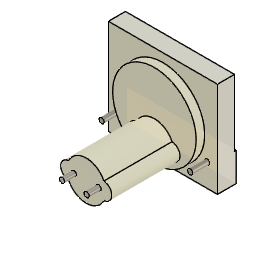
cpu usage panel v51 (Autodesk Fusion 360 archive; units mm, degrees)
design "galvanometer"
Autodesk Fusion 360 part; units mm, degrees
sketch "Sketch1" plane through (0, 0, 0) normal (0, 1, 0) x (1, 0, 0)
  line L0 (32, -28) -> (-32, -28)
  line L1 (-32, -28) -> (-32, 28)
  line L2 (-32, 28) -> (32, 28)
  line L3 (32, 28) -> (32, -28)
  line L4 (32, -28) -> (-32, 28) construction
  circle A0 centre (0, 1.5) radius 24.5
  line L5 (0, 1.5) -> (0, 0) construction
  line L6 (26, 14.5) -> (-26, 14.5) construction
  line L7 (0, 0) -> (0, 14.5) construction
  circle A1 centre (-26, 14.5) radius 1.5
  line L8 (32, 11) -> (-32, 11)
  circle A2 centre (0, 14.5) radius 11.5
  circle A3 centre (-7.25, 14.5) radius 1.5
  circle A4 centre (-10, 14.5) radius 5
  circle A5 centre (26, 14.5) radius 1.5
  circle A6 centre (10, 14.5) radius 5
  circle A7 centre (7.25, 14.5) radius 1.5
  dimension "d1" = 64
  dimension "d2" = 56
  dimension "d3" = 49
  dimension "d4" = 1.5
  dimension "d5" = 52
  dimension "d6" = 14.5
  dimension "d7" = 3
  dimension "d14" = 17
  dimension "d18" = 23
  dimension "d19" = 3
  dimension "d20" = 7.25
  dimension "d26" = 10
  dimension "d27" = 10
  constraint horizontal L0
  constraint vertical L1
  constraint horizontal L2
  constraint vertical L3
  constraint midpoint L5.end L4
  constraint coincident A0.centre L5.start
  constraint coincident L5.end L7.start
  constraint vertical L5
  constraint horizontal L6
  constraint perpendicular L6 L7
  constraint midpoint L6 L7.end
  constraint coincident L6.end A1.centre
  constraint coincident L3 L8.start
  constraint coincident L1 L8.end
  constraint perpendicular L1 L8
  constraint coincident L7 A2.centre
  constraint coincident L7.end A2.centre
  constraint coincident L6 A3.centre
  constraint symmetric L7 A1 A5
  constraint symmetric L7 A3 A7
  constraint symmetric L7 A4 A6
  constraint coincident L6 A4.centre
  measures "d1" distance of L0.start L0.end
  measures "d2" distance of L0.end L1.end
  measures "d3" diameter of A0
  measures "d4" distance of L5.end A0.centre
  measures "d5" distance of L6.start L6.end
  measures "d6" distance of L5.end L7.end
  measures "d7" diameter of A1
  measures "d14" distance of L2 L8
  measures "d18" diameter of A2
  measures "d19" diameter of A3
  measures "d20" distance of L7.end A3.centre
  measures "d26" diameter of A4
  measures "d27" distance of L7.end A4.centre
extrude "Extrude1" add sketch "Sketch1" along normal blind 10 contours L0 L1 L3 A0 L8 | L1 L2 L3 A0 L8 | A0 L8 A2 A6 | A0 L8 A2 A4 A6 | A0 L8 A2 A4 | L8 A2 A4 A6 | L8 A2 A6 | L8 A2 A6 | L8 A2 A4 | L8 A2 A4 | L8 A2 A6 | L8 A2 A4 | L8 A2 A6 | L8 A2 A4 A6 | L8 A2 A4 | A1 | A3 | A5 | A7 makes body 1
extrude "Extrude4" add sketch "Sketch1" along normal blind 1 from surface at 10 contours L1 L2 L3 A0 L8 | A0 L8 A2 A6 | A0 L8 A2 A4 | L8 A2 A4 A6 | L8 A2 A6 | L8 A2 A4 | L8 A2 A6 | L8 A2 A4 | A1 | A3 | A5 | A7 picked at (0.0435, 19.8621) picked at (12.5496, 15.563) picked at (-12.6463, 14.6782) picked at (9.085, 17.6254) picked at (-9.0246, 17.6974) bodies 1
extrude "Extrude2" add sketch "Sketch1" against normal blind 5 separate body contours A0 L8 A2 A6 | A0 L8 A2 A4 A6 | A0 L8 A2 A4 | L8 A2 A4 A6 | L8 A2 A6 | L8 A2 A6 | L8 A2 A4 | L8 A2 A4 | L8 A2 A6 | L8 A2 A4 | L8 A2 A6 | L8 A2 A4 A6 | L8 A2 A4 | A3 | A7 makes body 2
extrude "Extrude3" add sketch "Sketch1" against normal blind 10 contours A1 | A5 bodies 1 2
extrude "Extrude5" add sketch "Sketch1" against normal blind 45 contours L8 A2 A4 A6 | L8 A2 A6 | L8 A2 A6 | L8 A2 A4 | L8 A2 A4 | L8 A2 A6 | L8 A2 A4 | L8 A2 A6 | L8 A2 A4 A6 | L8 A2 A4 | A3 | A7 bodies 1 2
extrude "Extrude6" add sketch "Sketch1" against normal blind 7 from surface at -45 contours A3 | A7 bodies 1
equation "d20 = ( 14.5 / 2 ) * 1 mm"
named bodies: "galvanometer"
